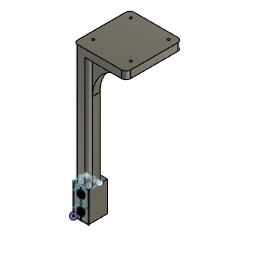
Sovol SV05 90 degree spool holder mount v2 (Autodesk Fusion 360 design; units mm, degrees)
Autodesk Fusion 360 part; units mm, degrees
note: some values were not read from the file. Set by a fixed rule: which sketch regions a step uses.
sketch "Sketch1" plane through (0, 0, 0) normal (0, 1, 0) x (1, 0, 0)
  line L0 (0, 0) -> (20, 0)
  line L1 (20, 0) -> (20, -40)
  line L2 (20, -40) -> (0, -40)
  line L3 (0, -40) -> (0, 0)
  line L4 (20, -40) -> (10, -40)
  line L5 (10, -40) -> (10, 0)
  line L6 (10, -40) -> (10, -30)
  line L7 (10, 0) -> (10, -10)
  circle A0 centre (10, -10) radius 2.75
  circle A1 centre (10, -30) radius 2.75
  circle A2 centre (10, -30) radius 4.75
  circle A3 centre (10, -10) radius 4.75
  dimension "d1" = 20
  dimension "d2" = 40
  dimension "d3" = 10
  dimension "d4" = 10
  dimension "d5" = 10
  dimension "d6" = 5.5
  dimension "d7" = 5.5
  dimension "d10" = 9.5
  dimension "d11" = 9.5
  constraint horizontal L0
  constraint vertical L1
  constraint horizontal L2
  constraint vertical L3
  constraint coincident L0.start L3.end
  constraint perpendicular L1 L4
  constraint midpoint L0 L5.end
  constraint perpendicular L2 L6
  constraint parallel L5 L7
  constraint coincident L7.end A0.centre
  constraint coincident L6.end A1.centre
  constraint concentric A1 A2
  constraint concentric A0 A3
  measures "d1" distance of L0.start L0.end
  measures "d2" distance of L0.start L2.end
  measures "d3" distance of L1.end L4.end
  measures "d4" distance of L4.end L6.end
  measures "d5" distance of L5.end L7.end
  measures "d6" diameter of A0
  measures "d7" diameter of A1
  measures "d10" diameter of A2
  measures "d11" diameter of A3
extrude "Extrude1" add sketch "Sketch1" along normal blind 25 contours L0 L2 L3 L5 L6 L7 A2 A3 | L0 L1 L2 L4 L5 L6 L7 A2 A3 | L5 L7 A0 A3 | L5 L7 A0 A3 | L5 L6 A1 A2 | L5 L6 A1 A2
extrude "Extrude2" cut sketch "Sketch1" along normal blind 10 contours L5 L7 A0 A3 | L5 L7 A0 A3 | L5 L6 A1 A2 | L5 L6 A1 A2
sketch "Sketch2" plane through (0, 0, 0) normal (1, 0, 0) x (0, 1, 0)
  line L0 (0, 0) -> (20, 0)
  line L1 (20, 0) -> (20, 40)
  line L2 (20, 40) -> (0, 40)
  line L3 (0, 40) -> (0, 0)
  line L4 (0, 30) -> (10, 30)
  line L5 (0, 10) -> (10, 10)
  circle A0 centre (10, 30) radius 2.35
  circle A1 centre (10, 10) radius 2.35
  dimension "d14" = 20
  dimension "d15" = 10
  dimension "d16" = 10
  dimension "d17" = 4.7
  dimension "d18" = 4.7
  constraint horizontal L0
  constraint vertical L1
  constraint horizontal L2
  constraint vertical L3
  constraint coincident L0.start L3.end
  constraint coincident L3 L4.start
  constraint perpendicular L3 L4
  constraint coincident L3 L5.start
  constraint perpendicular L3 L5
  constraint coincident L4.end A0.centre
  constraint coincident L5.end A1.centre
  measures "d14" distance of L0.start L0.end
  measures "d15" distance of L4.start L4.end
  measures "d16" distance of L5.start L5.end
  measures "d17" diameter of A0
  measures "d18" diameter of A1
sketch "Sketch3" plane through (0, 0, 40) normal (0, 0, 1) x (-1, 0, 0)
  line L0 (0, 0) -> (-20, 0)
  line L1 (-20, 0) -> (-20, -25)
  line L2 (-20, -25) -> (0, -25)
  line L3 (0, -25) -> (0, 0)
  line L4 (-15, 0) -> (-5, 0)
  line L5 (0, -5) -> (0, -15.3305)
  line L6 (-20, -15.3305) -> (-20, -5)
  line L7 (-10.403, -10.0836) -> (-9.4234, -10.0836)
  line L8 (0, -10) -> (0, -15.3305)
  line L9 (-19, -16.3305) -> (-15.6115, -16.3305)
  line L10 (-14.6115, -15.3305) -> (-14.6115, -12.2318)
  line L11 (-1, -16.3305) -> (-4.0034, -16.3305)
  line L12 (-5.0034, -15.3305) -> (-5.0034, -12.4938)
  arc A0 (-5.0034, -12.4938) -> (-14.6115, -12.2318) centre (-9.9132, -16.2396) ccw
  line L13 (-1, -16.3305) -> (-4.0034, -16.3305)
  line L14 (-15.6115, -16.3305) -> (-19, -16.3305)
  line L15 (-1, -16.3305) -> (-4.0034, -16.3305)
  line L16 (-15.6115, -16.3305) -> (-19, -16.3305)
  arc A1 (-15.6115, -16.3305) -> (-14.6115, -15.3305) centre (-15.6115, -15.3305) ccw
  arc A2 (-5.0034, -15.3305) -> (-4.0034, -16.3305) centre (-4.0034, -15.3305) ccw
  arc A3 (-20, -15.3305) -> (-19, -16.3305) centre (-19, -15.3305) ccw
  arc A4 (-1, -16.3305) -> (0, -15.3305) centre (-1, -15.3305) ccw
  arc A5 (-15, 0) -> (-20, -5) centre (-15, -5) ccw
  arc A6 (0, -5) -> (-5, 0) centre (-5, -5) ccw
  dimension "d24" = 1
  dimension "d25" = 1
  dimension "d26" = 5
  constraint horizontal L4
  constraint vertical L5
  constraint horizontal L15
  constraint vertical L6
  constraint horizontal L13
  constraint horizontal L7
  constraint vertical L8
  constraint horizontal L9
  constraint vertical L10
  constraint horizontal L11
  constraint vertical L12
  constraint collinear L13 L14
  constraint collinear L15 L16
  constraint coincident A0 L7.end
  constraint coincident A0 L7.start
  constraint tangent L9 A1
  constraint tangent L10 A1
  constraint tangent L12 A2
  constraint tangent L15 A2
  constraint equal A1 A2
  constraint tangent L6 A3
  constraint tangent L14 A3
  constraint tangent L13 A4
  constraint tangent L8 A4
  constraint equal A3 A4
  constraint tangent L6 A5
  constraint tangent L4 A5
  constraint tangent L4 A6
  constraint tangent L5 A6
  constraint equal A5 A6
  measures "d24" radius of A1
  measures "d25" radius of A3
  measures "d26" radius of A5
extrude "Extrude4" add sketch "Sketch3" along normal blind 150 contours L0 L1 L3 L4 L5 L6 L8 L9 L10 L11 L12 A0 L13 L14 L15 L16 A1 A2 A3 A4 A5 A6
sketch "Sketch4" plane through (0, 0, 190) normal (0, 0, 1) x (-1, 0, 0)
  line L0 (0, -15.3305) -> (0, -5)
  arc A0 (0, -5) -> (-5, 0) centre (-5, -5) ccw
  line L1 (-5, 0) -> (-15, 0)
  arc A1 (-15, 0) -> (-20, -5) centre (-15, -5) ccw
  line L2 (-20, -5) -> (-20, -15.3305)
  arc A2 (-20, -15.3305) -> (-19, -16.3305) centre (-19, -15.3305) ccw
  line L3 (-19, -16.3305) -> (-15.6115, -16.3305)
  arc A3 (-15.6115, -16.3305) -> (-14.6115, -15.3305) centre (-15.6115, -15.3305) ccw
  line L4 (-14.6115, -15.3305) -> (-14.6115, -12.2318)
  arc A4 (-5.0034, -12.4938) -> (-14.6115, -12.2318) centre (-9.9132, -16.2396) ccw
  line L5 (-5.0034, -12.4938) -> (-5.0034, -15.3305)
  arc A5 (-5.0034, -15.3305) -> (-4.0034, -16.3305) centre (-4.0034, -15.3305) ccw
  line L6 (-4.0034, -16.3305) -> (-1, -16.3305)
  arc A6 (-1, -16.3305) -> (0, -15.3305) centre (-1, -15.3305) ccw
  circle A7 centre (-9.9132, -16.2396) radius 1.55
  line L7 (0, 0) -> (-63.7918, 0)
  line L8 (-69.7918, -6) -> (-69.7918, -68.86)
  line L9 (-63.7918, -74.86) -> (-6, -74.86)
  line L10 (0, -68.86) -> (0, 0)
  arc A8 (-63.7918, 0) -> (-69.7918, -6) centre (-63.7918, -6) ccw
  arc A9 (-69.7918, -68.86) -> (-63.7918, -74.86) centre (-63.7918, -68.86) ccw
  arc A10 (-6, -74.86) -> (0, -68.86) centre (-6, -68.86) ccw
  arc A11 (0, -5) -> (-5, 0) centre (-5, -5) ccw
  circle A12 centre (-59.9132, -16.2396) radius 1.55
  circle A13 centre (-60, -66.2375) radius 1.55
  circle A14 centre (-9.9132, -66.2396) radius 1.55
  dimension "d29" = 3.1
  dimension "d30" = 50
  dimension "d31" = 50
  dimension "d32" = 6
  dimension "d33" = 3.1
  dimension "d34" = 3.1
  dimension "d35" = 3.1
  constraint concentric A4 A7
  constraint horizontal L7
  constraint vertical L8
  constraint horizontal L9
  constraint vertical L10
  constraint coincident L7.start L10.end
  constraint tangent L8 A8
  constraint tangent L7 A8
  constraint tangent L8 A9
  constraint tangent L9 A9
  constraint equal A8 A9
  constraint tangent L9 A10
  constraint tangent L10 A10
  constraint equal A8 A10
  measures "d29" diameter of A7
  measures "d30" distance of A4.centre A12.centre
  measures "d31" distance of A4.centre A14.centre
  measures "d32" radius of A8
  measures "d33" diameter of A12
  measures "d34" diameter of A13
  measures "d35" diameter of A14
extrude "Extrude5" add sketch "Sketch4" along normal blind 10 contours L0 A0 L1 A1 L2 A2 L3 A3 L4 A4 L5 A5 L6 A6 L7 L10 A11 | A1 L2 A2 L3 A3 L4 A4 L5 A5 L6 A6 L7 L8 L9 L10 A8 A9 A10
sketch "Sketch5" plane through (0, 0, 0) normal (0, -1, 0) x (1, 0, 0)
  circle A0 centre (10, 30) radius 4.75
  circle A1 centre (10, 10) radius 4.75
  line L0 (20, 0) -> (20, 40)
  line L1 (20, 40) -> (15, 40)
  line L2 (15, 40) -> (15, 190)
  line L3 (15, 190) -> (63.7918, 190)
  line L4 (63.7918, 190) -> (63.7918, 200)
  line L5 (63.7918, 200) -> (5, 200)
  line L6 (5, 200) -> (5, 40)
  line L7 (5, 40) -> (0, 40)
  line L8 (0, 40) -> (0, 0)
  line L9 (0, 0) -> (20, 0)
  line L10 (20, 190) -> (65, 190)
  line L11 (20, 145) -> (20, 190)
  arc A2 (65, 190) -> (20, 145) centre (65, 145) ccw
  constraint horizontal L10
  constraint vertical L11
  constraint coincident L3 L10.start
extrude "Extrude6" add sketch "Sketch5" against normal blind 10 from surface at -5 contours L3 L10 L11 A2
extrude "Extrude7" cut 1 faces at (59.9434, 14.7871, 190) along direction (0, 0, -1) blind 5
